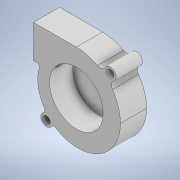
# Autodesk Inventor part: 5015 RADIAL FAN
Saved by Autodesk Inventor 2022 (Build 260153070, 153G)
## iProperties
Created: 2022-01-01
Part Number: 5015 RADIAL FAN
Material: Generic
Document SubType Name: Modeling
Designer: a laptop
Density: 1 g/cm^3
Appearance: Default
Author: a laptop
Autodesk Inventor part; units mm, degrees
ref_plane "YZ Plane" through (0, 0, 0) normal (1, 0, 0) x (0, 1, 0)
ref_plane "XZ Plane" through (0, 0, 0) normal (0, 1, 0) x (-1, 0, 0)
ref_plane "XY Plane" through (0, 0, 0) normal (0, 0, 1) x (1, 0, 0)
sketch "Sketch1" plane through (0, 0, 0) normal (0, 0, 1) x (1, 0, 0)
  line L0 (-25.6, 26.3) -> (-25.6, 6.6)
  line L1 (-25.6, 26.3) -> (0, 26.3)
  line L2 (0, 26.3) -> (0, 0) construction
  line L3 (0, 0) -> (26.3, 0)
  arc A0 (26.3, 0) -> (21.4915, 15.1594) centre (0, 0) ccw
  line L4 (-25.6, 6.6) -> (-23.6, 6.6)
  circle A1 centre (-17.8, -20.3) radius 2.25
  arc A2 (0.8, -25.5) -> (26.3, 0) centre (0.8, 0) ccw
  line L5 (-6.4086, -25.5) -> (23, -25.5) construction
  arc A3 (-22.1547, 4.6986) -> (-23.6, 6.6) centre (-23.6, 5.1) ccw
  circle A4 centre (20.3, 22.8) radius 2.25
  arc A5 (-22.1547, 4.6986) -> (-19.151, -14.6964) centre (0.8, -1.6765) ccw
  arc A6 (-19.7128, -17.3689) -> (-19.151, -14.6964) centre (-20.7682, -15.7518) ccw
  arc A7 (-12.1947, -21.6439) -> (-14.8665, -22.2091) centre (-13.248, -23.2624) ccw
  arc A8 (-19.7128, -17.3689) -> (-14.8665, -22.2091) centre (-17.8, -20.3) ccw
  arc A9 (-12.1947, -21.6439) -> (0.8, -25.5) centre (0.8, -1.6765) ccw
  arc A10 (22.3174, 19.9399) -> (17.2258, 24.4732) centre (20.3, 22.8) ccw
  arc A11 (12.5728, 23.1001) -> (17.2258, 24.4732) centre (14.2128, 26.1131) ccw
  arc A12 (22.3174, 19.9399) -> (21.4915, 15.1594) centre (24.2947, 17.1367) ccw
  arc A13 (12.5728, 23.1001) -> (0, 26.3) centre (0, 0) ccw
  dimension "d1" = 25.6
  dimension "d2" = 19.7
  dimension "d6" = 4.5
  dimension "d8" = 17.8
  dimension "d9" = 26.3
  dimension "d10" = 51.8
  dimension "d11" = 20.3
  dimension "d12" = 1.5
  dimension "d13" = 4.5
  dimension "d14" = 22.8
  dimension "d15" = 20.3
  dimension "d16" = 2
  dimension "d18" = 90
  dimension "d19" = 90
  dimension "d20" = 1.25
  dimension "d21" = 1.25
  dimension "d22" = 90
  dimension "d23" = 90
  constraints: 25 point on circle, 16 tangent, 14 centre point, 12 end point, 3 coincident, 3 perpendicular, 2 horizontal, 1 parallel, 1 point on line, 1 vertical
  measures "d1" distance of L0.start L1.end
  measures "d2" distance of L0.start L0.end
  measures "d6" diameter of A1
  measures "d8" distance from line of L2 A1.centre
  measures "d9" distance of L1.end L2.end
  measures "d10" distance from line of L1.end L5
  measures "d11" vertical distance of point (0, 0) A1.centre
  measures "d12" radius of A3
  measures "d13" diameter of A4
  measures "d14" vertical distance of point (0, 0) A4.centre
  measures "d15" horizontal distance of A4.centre point (0, 0)
  measures "d16" horizontal distance of A3.centre L0.end
  measures "d20" radial gap between concentric circles of A8 A1
  measures "d21" radial gap between concentric circles of A4 A10
extrude "Extrusion1" add sketch "Sketch1" along normal blind 15.6
sketch "Sketch2" plane through (-25.6, 6.6, 0) normal (-1, 0, 0) x (0, 0, 1)
  line L0 (1.7, 18.25) -> (14.3, 18.25)
  line L1 (14.3, 18.25) -> (14.3, 1.15)
  line L2 (14.3, 1.15) -> (1.7, 1.15)
  line L3 (1.7, 1.15) -> (1.7, 18.25)
  point P0 (0, -6.6)
  point P1 (0, 19.7)
  dimension "d26" = 12.6
  dimension "d27" = 17.1
  dimension "d28" = 1.7
  dimension "d29" = 1.45
  constraints: 8 end point, 2 parallel, 1 horizontal, 1 perpendicular
  measures "d26" distance of L0.start L0.end
  measures "d27" distance of L0.end L1.end
  measures "d28" distance from line of point (0, 19.7) L3
  measures "d29" vertical distance of point (0, 19.7) L0.start
extrude "Extrusion2" cut sketch "Sketch2" against normal blind 15.6
sketch "Sketch3" plane through (0, 0, 15.6) normal (0, 0, 1) x (1, 0, 0)
  circle A0 centre (0, 0) radius 16
  dimension "d32" = 32
  constraints: 1 centre point, 1 coincident
  measures "d32" diameter of A0
extrude "Extrusion3" cut sketch "Sketch3" against normal blind 13.9
body "Solid1"
